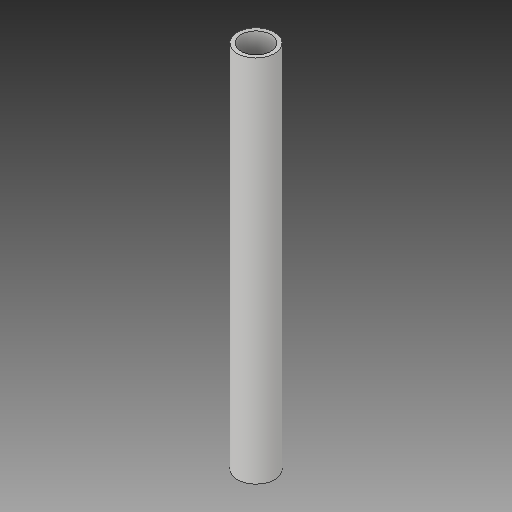
# Autodesk Inventor part: BearingsSpacer
Saved by Autodesk Inventor 2019.2 (Build 232265000, 265)
## iProperties
Created: 2018-01-25
Part Number: BearingsSpacer
Material: Generic
Document SubType Name: Modeling
Designer: eroldan
Density: 1 g/cm^3
Appearance: Default
Author: eroldan
Autodesk Inventor part; units mm, degrees
ref_plane "YZ Plane" through (0, 0, 0) normal (1, 0, 0) x (0, 1, 0)
ref_plane "XZ Plane" through (0, 0, 0) normal (0, 1, 0) x (-1, 0, 0)
ref_plane "Work Plane2" through (86.3313, -0.6, -206.3) normal (0, -1, 0) x (0.4516, 0, -0.8922)
sketch "Sketch2" plane through (86.3313, -0.6, -206.3) normal (0, -1, 0) x (0.4516, 0, -0.8922)
  circle A0 centre (0, -10) radius 15 construction
  circle A1 centre (0, -10) radius 7.9375
  circle A2 centre (0, -10) radius 6.3375
  point P0 (-223.0522, 16.1405)
  dimension "d4" = 15.875
  dimension "d5" = 1.6
  constraints: 2 centre point, 1 coincident
  measures "d4" diameter of A1
  measures "d5" radial gap between concentric circles of A1 A2
extrude "Extrusion2" add sketch "Sketch2" along normal mid plane 158
body "Solid2"
